Autodesk Inventor part; units mm, degrees
(part 4 of 5)
  arc A1516 (16.6024, 15.6098) -> (16.5463, 15.6184) centre (16.5463, 15.4301) ccw
  arc A1517 (16.6393, 15.5846) -> (16.6024, 15.6098) centre (16.5796, 15.5369) ccw
  arc A1518 (16.6599, 15.5394) -> (16.6393, 15.5846) centre (16.56, 15.5212) ccw
  arc A1519 (16.6663, 15.4684) -> (16.6599, 15.5394) centre (16.2689, 15.4684) ccw
  arc A1520 (16.6599, 14.6174) -> (16.6663, 14.6884) centre (16.2689, 14.6884) ccw
  arc A1521 (16.6393, 14.5721) -> (16.6599, 14.6174) centre (16.56, 14.6356) ccw
  arc A1522 (16.6024, 14.547) -> (16.6393, 14.5721) centre (16.5796, 14.6199) ccw
  arc A1523 (16.5463, 14.5384) -> (16.6024, 14.547) centre (16.5463, 14.7267) ccw
  arc A1524 (16.4902, 14.547) -> (16.5463, 14.5384) centre (16.5463, 14.7267) ccw
  arc A1525 (16.4533, 14.5721) -> (16.4902, 14.547) centre (16.5129, 14.6199) ccw
  arc A1526 (16.4327, 14.6174) -> (16.4533, 14.5721) centre (16.5325, 14.6356) ccw
  arc A1527 (16.4263, 14.6884) -> (16.4327, 14.6174) centre (16.8237, 14.6884) ccw
  arc A1528 (16.4327, 14.7594) -> (16.4263, 14.6884) centre (16.8237, 14.6884) ccw
  arc A1529 (16.4533, 14.8046) -> (16.4327, 14.7594) centre (16.5325, 14.7412) ccw
  arc A1530 (16.4902, 14.8298) -> (16.4533, 14.8046) centre (16.5129, 14.7569) ccw
  arc A1531 (16.5463, 14.8384) -> (16.4902, 14.8298) centre (16.5463, 14.6501) ccw
  arc A1532 (16.6024, 14.8298) -> (16.5463, 14.8384) centre (16.5463, 14.6501) ccw
  arc A1533 (16.6393, 14.8046) -> (16.6024, 14.8298) centre (16.5796, 14.7569) ccw
  arc A1534 (16.6599, 14.7594) -> (16.6393, 14.8046) centre (16.56, 14.7412) ccw
  arc A1535 (16.6663, 14.6884) -> (16.6599, 14.7594) centre (16.2689, 14.6884) ccw
  arc A1536 (16.6306, 13.7177) -> (16.6363, 13.8142) centre (15.8065, 13.8142) ccw
  arc A1537 (16.6121, 13.6524) -> (16.6306, 13.7177) centre (16.4198, 13.7424) ccw
  arc A1538 (16.5793, 13.6115) -> (16.6121, 13.6524) centre (16.5112, 13.6997) ccw
  arc A1539 (16.5313, 13.5898) -> (16.5793, 13.6115) centre (16.5098, 13.7014) ccw
  arc A1540 (16.4797, 13.5909) -> (16.5313, 13.5898) centre (16.508, 13.7107) ccw
  arc A1541 (16.4475, 13.615) -> (16.4797, 13.5909) centre (16.4913, 13.64) ccw
  arc A1542 (16.4306, 13.6695) -> (16.4475, 13.615) centre (16.5623, 13.6804) ccw
  arc A1543 (16.4263, 13.774) -> (16.4306, 13.6695) centre (17.6884, 13.774) ccw
  arc A1544 (16.4293, 13.8553) -> (16.4263, 13.774) centre (17.5205, 13.774) ccw
  arc A1545 (16.4384, 13.9305) -> (16.4293, 13.8553) centre (17.2504, 13.7941) ccw
  arc A1546 (16.4515, 13.9917) -> (16.4384, 13.9305) centre (17.1328, 13.8139) ccw
  arc A1547 (16.4675, 14.0196) -> (16.4515, 13.9917) centre (16.5111, 13.9761) ccw
  arc A1548 (16.5292, 14.0474) -> (16.4675, 14.0196) centre (16.5349, 13.9523) ccw
  arc A1549 (16.5849, 14.0231) -> (16.5292, 14.0474) centre (16.5332, 13.9806) ccw
  arc A1550 (16.6239, 13.9404) -> (16.5849, 14.0231) centre (16.4401, 13.9041) ccw
  arc A1551 (16.6363, 13.8142) -> (16.6239, 13.9404) centre (15.9849, 13.8142) ccw
  arc A1552 (5.9121, 15.2297) -> (5.9567, 15.3581) centre (3.0245, 16.304) ccw
  arc A1553 (5.8608, 15.0999) -> (5.9121, 15.2297) centre (2.705, 16.4228) ccw
  arc A1554 (5.8104, 14.9862) -> (5.8608, 15.0999) centre (3.0618, 16.2733) ccw
  arc A1555 (5.7705, 14.914) -> (5.8104, 14.9862) centre (5.2469, 15.2501) ccw
  arc A1556 (5.7705, 14.914) -> (5.7251, 14.8316) centre (6.3667, 14.5314) ccw
  arc A1557 (5.7251, 14.8316) -> (5.7257, 14.7867) centre (5.7719, 14.8097) ccw
  arc A1558 (5.7257, 14.7867) -> (5.7624, 14.7497) centre (5.8002, 14.8239) ccw
  arc A1559 (5.7624, 14.7497) -> (5.8803, 14.6939) centre (6.7561, 16.6973) ccw
  arc A1560 (5.9708, 14.6449) -> (5.8803, 14.6939) centre (5.6348, 14.1324) ccw
  arc A1561 (5.9663, 14.6196) -> (5.9708, 14.6449) centre (5.9631, 14.6332) ccw
  arc A1562 (5.8708, 14.6078) -> (5.9663, 14.6196) centre (5.8638, 15.0599) ccw
  arc A1563 (5.4913, 14.6033) -> (5.8708, 14.6078) centre (5.0515, 67.172) ccw
  line L488 (5.4913, 14.6033) -> (4.9063, 14.5984)
  line L489 (4.9063, 14.5984) -> (4.9063, 13.4884)
  line L490 (4.9063, 13.4884) -> (4.9063, 12.3784)
  line L491 (4.9063, 12.3784) -> (5.1727, 12.3784)
  arc A1564 (5.1727, 12.3784) -> (5.2775, 12.3828) centre (5.1727, 13.6312) ccw
  arc A1565 (5.2775, 12.3828) -> (5.3718, 12.396) centre (5.206, 13.235) ccw
  arc A1566 (5.3718, 12.396) -> (5.4463, 12.4151) centre (5.2366, 13.0801) ccw
  arc A1567 (5.4463, 12.4151) -> (5.4763, 12.4384) centre (5.4299, 12.4671) ccw
  arc A1568 (5.5036, 12.4616) -> (5.4763, 12.4384) centre (5.5257, 12.4079) ccw
  arc A1569 (5.5621, 12.4808) -> (5.5036, 12.4616) centre (5.6655, 12.0669) ccw
  arc A1570 (5.6359, 12.494) -> (5.5621, 12.4808) centre (5.6964, 11.9435) ccw
  arc A1571 (5.7163, 12.4984) -> (5.6359, 12.494) centre (5.7163, 11.7626) ccw
  arc A1572 (5.7967, 12.494) -> (5.7163, 12.4984) centre (5.7163, 11.7626) ccw
  arc A1573 (5.8705, 12.4808) -> (5.7967, 12.494) centre (5.7362, 11.9435) ccw
  arc A1574 (5.9289, 12.4616) -> (5.8705, 12.4808) centre (5.767, 12.0669) ccw
  arc A1575 (5.9563, 12.4384) -> (5.9289, 12.4616) centre (5.9069, 12.4079) ccw
  arc A1576 (5.9563, 12.4384) -> (5.9863, 12.4151) centre (6.0027, 12.4671) ccw
  arc A1577 (5.9863, 12.4151) -> (6.0607, 12.396) centre (6.196, 13.0801) ccw
  arc A1578 (6.0607, 12.396) -> (6.1551, 12.3828) centre (6.2266, 13.235) ccw
  arc A1579 (6.1551, 12.3828) -> (6.2598, 12.3784) centre (6.2598, 13.6312) ccw
  line L492 (6.2598, 12.3784) -> (6.5263, 12.3784)
  line L493 (6.5263, 12.3784) -> (6.5263, 13.4884)
  line L494 (6.5263, 13.4884) -> (6.5263, 14.5984)
  line L495 (6.5263, 14.5984) -> (6.385, 14.5984)
  line L496 (6.385, 14.5984) -> (6.2438, 14.5984)
  line L497 (6.2438, 14.5984) -> (6.3805, 14.8841)
  arc A1580 (6.3805, 14.8841) -> (6.4343, 15.0063) centre (4.4938, 15.787) ccw
  arc A1581 (6.4343, 15.0063) -> (6.4828, 15.1374) centre (4.1091, 15.9418) ccw
  arc A1582 (6.4828, 15.1374) -> (6.52, 15.2583) centre (4.3654, 15.8549) ccw
  arc A1583 (6.52, 15.2583) -> (6.5368, 15.3451) centre (5.9846, 15.4066) ccw
  arc A1584 (6.5368, 15.3451) -> (6.5386, 15.4464) centre (5.9904, 15.4059) ccw
  arc A1585 (6.5386, 15.4464) -> (6.5135, 15.5043) centre (6.4433, 15.4394) ccw
  arc A1586 (6.5135, 15.5043) -> (6.4513, 15.5459) centre (6.3953, 15.395) ccw
  arc A1587 (6.4513, 15.5459) -> (6.3064, 15.5941) centre (5.6805, 13.471) ccw
  line L498 (6.3064, 15.5941) -> (6.0566, 15.6678)
  line L499 (6.0566, 15.6678) -> (5.9567, 15.3581)
  arc A1588 (5.9784, 13.8303) -> (5.9863, 13.9384) centre (5.2368, 13.9384) ccw
  arc A1589 (5.9488, 13.7834) -> (5.9784, 13.8303) centre (5.9109, 13.8402) ccw
  arc A1590 (5.8854, 13.7625) -> (5.9488, 13.7834) centre (5.8793, 13.8876) ccw
  arc A1591 (5.7163, 13.7584) -> (5.8854, 13.7625) centre (5.7163, 17.2389) ccw
  arc A1592 (5.5472, 13.7625) -> (5.7163, 13.7584) centre (5.7163, 17.2389) ccw
  arc A1593 (5.4838, 13.7834) -> (5.5472, 13.7625) centre (5.5533, 13.8876) ccw
  arc A1594 (5.4541, 13.8303) -> (5.4838, 13.7834) centre (5.5216, 13.8402) ccw
  arc A1595 (5.4463, 13.9384) -> (5.4541, 13.8303) centre (6.1958, 13.9384) ccw
  arc A1596 (5.4541, 14.0465) -> (5.4463, 13.9384) centre (6.1958, 13.9384) ccw
  arc A1597 (5.4838, 14.0934) -> (5.4541, 14.0465) centre (5.5216, 14.0366) ccw
  arc A1598 (5.5472, 14.1143) -> (5.4838, 14.0934) centre (5.5533, 13.9892) ccw
  arc A1599 (5.7163, 14.1184) -> (5.5472, 14.1143) centre (5.7163, 10.6379) ccw
  arc A1600 (5.8854, 14.1143) -> (5.7163, 14.1184) centre (5.7163, 10.6379) ccw
  arc A1601 (5.9488, 14.0934) -> (5.8854, 14.1143) centre (5.8793, 13.9892) ccw
  arc A1602 (5.9784, 14.0465) -> (5.9488, 14.0934) centre (5.9109, 14.0366) ccw
  arc A1603 (5.9863, 13.9384) -> (5.9784, 14.0465) centre (5.2368, 13.9384) ccw
  arc A1604 (5.9795, 12.9829) -> (5.9863, 13.0949) centre (5.0516, 13.0949) ccw
  arc A1605 (5.9519, 12.9387) -> (5.9795, 12.9829) centre (5.9186, 12.9902) ccw
  arc A1606 (5.8934, 12.9222) -> (5.9519, 12.9387) centre (5.8958, 13.0254) ccw
  arc A1607 (5.7313, 12.9299) -> (5.8934, 12.9222) centre (5.9734, 16.2763) ccw
  arc A1608 (5.5847, 12.9458) -> (5.7313, 12.9299) centre (5.8816, 15.0074) ccw
  arc A1609 (5.5151, 12.9725) -> (5.5847, 12.9458) centre (5.6086, 13.1122) ccw
  arc A1610 (5.4776, 13.0216) -> (5.5151, 12.9725) centre (5.5682, 13.0518) ccw
  arc A1611 (5.4573, 13.1134) -> (5.4776, 13.0216) centre (5.9087, 13.1653) ccw
  arc A1612 (5.4541, 13.212) -> (5.4573, 13.1134) centre (6.0551, 13.1822) ccw
  arc A1613 (5.4791, 13.2554) -> (5.4541, 13.212) centre (5.509, 13.2092) ccw
  arc A1614 (5.5401, 13.2748) -> (5.4791, 13.2554) centre (5.5452, 13.1534) ccw
  arc A1615 (5.7123, 13.2784) -> (5.5401, 13.2748) centre (5.7123, 9.1613) ccw
  arc A1616 (5.8852, 13.2743) -> (5.7123, 13.2784) centre (5.7123, 9.5941) ccw
  arc A1617 (5.9489, 13.2534) -> (5.8852, 13.2743) centre (5.8794, 13.1495) ccw
  arc A1618 (5.9786, 13.206) -> (5.9489, 13.2534) centre (5.9108, 13.1965) ccw
  arc A1619 (5.9863, 13.0949) -> (5.9786, 13.206) centre (5.1834, 13.0949) ccw
  arc A1620 (5.1763, 15.5756) -> (5.0533, 15.5279) centre (5.2917, 15.0958) ccw
  arc A1621 (5.0533, 15.5279) -> (4.9985, 15.4587) centre (5.1085, 15.428) ccw
  arc A1622 (4.9985, 15.4587) -> (4.9964, 15.3478) centre (5.2114, 15.3992) ccw
  arc A1623 (4.9964, 15.3478) -> (5.0551, 15.1421) centre (7.4152, 15.926) ccw
  line L500 (5.0551, 15.1421) -> (5.1571, 14.835)
  line L501 (5.1571, 14.835) -> (5.3767, 14.8746)
  arc A1624 (5.3767, 14.8746) -> (5.4626, 14.8914) centre (4.8255, 17.9263) ccw
  arc A1625 (5.4626, 14.8914) -> (5.539, 14.909) centre (5.0517, 16.8488) ccw
  arc A1626 (5.539, 14.909) -> (5.6021, 14.9258) centre (4.9452, 17.2724) ccw
  arc A1627 (5.6021, 14.9258) -> (5.6209, 14.936) centre (5.5891, 14.9722) ccw
  arc A1628 (5.6209, 14.936) -> (5.6282, 14.9553) centre (5.6064, 14.9526) ccw
  arc A1629 (5.6282, 14.9553) -> (5.6151, 15.0484) centre (2.1377, 14.5092) ccw
  arc A1630 (5.6151, 15.0484) -> (5.5949, 15.1599) centre (3.3594, 14.6987) ccw
  arc A1631 (5.5949, 15.1599) -> (5.5664, 15.2881) centre (1.5733, 14.3301) ccw
  arc A1632 (5.5664, 15.2881) -> (5.5061, 15.5023) centre (2.7572, 14.6142) ccw
  arc A1633 (5.5061, 15.5023) -> (5.4474, 15.5839) centre (5.3502, 15.4519) ccw
  arc A1634 (5.4474, 15.5839) -> (5.3578, 15.6077) centre (5.3723, 15.4819) ccw
  arc A1635 (5.3578, 15.6077) -> (5.1763, 15.5756) centre (5.5306, 14.1027) ccw
  arc A1636 (4.3963, 15.4254) -> (4.3262, 15.4003) centre (6.5047, 9.4466) ccw
  arc A1637 (4.3262, 15.4003) -> (4.2648, 15.3772) centre (5.6457, 11.7944) ccw
  arc A1638 (4.2648, 15.3772) -> (4.213, 15.357) centre (6.5581, 9.4269) ccw
  arc A1639 (4.213, 15.357) -> (4.2015, 15.3504) centre (4.2301, 15.3138) ccw
  arc A1640 (4.2015, 15.3504) -> (4.1907, 15.3135) centre (4.2217, 15.3244) ccw
  arc A1641 (4.1907, 15.3135) -> (4.2846, 15.0531) centre (22.7751, 21.87) ccw
  arc A1642 (4.2846, 15.0531) -> (4.3805, 14.801) centre (16.5632, 19.5799) ccw
  arc A1643 (4.3805, 14.801) -> (4.4225, 14.7507) centre (4.477, 14.8389) ccw
  arc A1644 (4.4225, 14.7507) -> (4.5215, 14.7338) centre (4.493, 14.8648) ccw
  arc A1645 (4.5215, 14.7338) -> (4.7003, 14.7868) centre (4.2534, 15.9649) ccw
  arc A1646 (4.7003, 14.7868) -> (4.8621, 14.8621) centre (4.2659, 15.9319) ccw
  arc A1647 (4.8621, 14.8621) -> (4.8854, 14.9263) centre (4.8367, 14.9076) ccw
  arc A1648 (4.8691, 14.9718) -> (4.8854, 14.9263) centre (5.8374, 15.2916) ccw
  arc A1649 (4.8421, 15.0549) -> (4.8691, 14.9718) centre (13.9102, 17.9581) ccw
  arc A1650 (4.8115, 15.152) -> (4.8421, 15.0549) centre (14.7921, 18.2404) ccw
  arc A1651 (4.7811, 15.2522) -> (4.8115, 15.152) centre (15.9198, 18.5894) ccw
  arc A1652 (4.7811, 15.2522) -> (4.7226, 15.4152) centre (3.2292, 14.7872) ccw
  arc A1653 (4.7226, 15.4152) -> (4.665, 15.4742) centre (4.6187, 15.3715) ccw
  arc A1654 (4.665, 15.4742) -> (4.5792, 15.4814) centre (4.6118, 15.3562) ccw
  arc A1655 (4.5792, 15.4814) -> (4.3963, 15.4254) centre (5.1542, 13.2763) ccw
  line L502 (17.3863, 11.5084) -> (17.3863, 11.3584)
  line L503 (17.3863, 11.3584) -> (16.6063, 11.3584)
  line L504 (16.6063, 11.3584) -> (15.8263, 11.3584)
  line L505 (15.8263, 11.3584) -> (15.8263, 10.8784)
  line L506 (15.8263, 10.8784) -> (15.8263, 10.3984)
  line L507 (15.8263, 10.3984) -> (16.1263, 10.3984)
  arc A1656 (16.1263, 10.3984) -> (16.3183, 10.4021) centre (16.1263, 15.337) ccw
  arc A1657 (16.3183, 10.4021) -> (16.3863, 10.4224) centre (16.3127, 10.545) ccw
  arc A1658 (16.3863, 10.4224) -> (16.4178, 10.4692) centre (16.352, 10.4795) ccw
  arc A1659 (16.4178, 10.4692) -> (16.4263, 10.5784) centre (15.718, 10.5784) ccw
  line L508 (16.4263, 10.5784) -> (16.4263, 10.7584)
  line L509 (16.4263, 10.7584) -> (16.7863, 10.7584)
  arc A1660 (17.0333, 10.7493) -> (16.7863, 10.7584) centre (16.7863, 7.3979) ccw
  arc A1661 (17.1238, 10.706) -> (17.0333, 10.7493) centre (17.0232, 10.612) ccw
  arc A1662 (17.1512, 10.6177) -> (17.1238, 10.706) centre (17.0463, 10.6336) ccw
  arc A1663 (17.1085, 10.4134) -> (17.1512, 10.6177) centre (15.2977, 10.8987) ccw
  arc A1664 (17.0633, 10.3374) -> (17.1085, 10.4134) centre (16.9508, 10.4557) ccw
  arc A1665 (16.9858, 10.2973) -> (17.0633, 10.3374) centre (16.9558, 10.4504) ccw
  arc A1666 (16.8319, 10.2813) -> (16.9858, 10.2973) centre (16.8197, 11.1452) ccw
  arc A1667 (16.4193, 10.2784) -> (16.8319, 10.2813) centre (16.4193, 39.5826) ccw
  line L510 (16.4193, 10.2784) -> (15.7663, 10.2784)
  line L511 (15.7663, 10.2784) -> (15.7663, 9.9784)
  line L512 (15.7663, 9.9784) -> (15.7663, 9.6784)
  line L513 (15.7663, 9.6784) -> (16.3063, 9.6784)
  arc A1668 (16.5317, 9.6744) -> (16.3063, 9.6784) centre (16.3063, 3.2633) ccw
  arc A1669 (16.7015, 9.6617) -> (16.5317, 9.6744) centre (16.4568, 7.5438) ccw
  arc A1670 (16.8239, 9.643) -> (16.7015, 9.6617) centre (16.5035, 7.9482) ccw
  arc A1671 (16.8463, 9.616) -> (16.8239, 9.643) centre (16.8188, 9.616) ccw
  arc A1672 (16.7656, 9.369) -> (16.8463, 9.616) centre (16.4279, 9.616) ccw
  arc A1673 (16.4245, 8.9438) -> (16.7656, 9.369) centre (11.8154, 12.9907) ccw
  arc A1674 (16.0426, 8.5495) -> (16.4245, 8.9438) centre (12.1999, 12.6532) ccw
  arc A1675 (15.7692, 8.3893) -> (16.0426, 8.5495) centre (15.5522, 9.0732) ccw
  arc A1676 (15.7692, 8.3893) -> (15.712, 8.3563) centre (15.8159, 8.2423) ccw
  arc A1677 (15.712, 8.3563) -> (15.7, 8.3129) centre (15.7404, 8.3251) ccw
  arc A1678 (15.7, 8.3129) -> (15.736, 8.2395) centre (15.9425, 8.3863) ccw
  arc A1679 (15.736, 8.2395) -> (15.8706, 8.0548) centre (23.8093, 13.9816) ccw
  arc A1680 (15.8706, 8.0548) -> (15.9586, 7.9412) centre (19.1235, 10.4833) ccw
  arc A1681 (15.9586, 7.9412) -> (16.0397, 7.8455) centre (17.8083, 9.427) ccw
  arc A1682 (16.0397, 7.8455) -> (16.1101, 7.7693) centre (18.4082, 9.9635) ccw
  arc A1683 (16.1101, 7.7693) -> (16.1357, 7.7584) centre (16.1357, 7.7938) ccw
  arc A1684 (16.1357, 7.7584) -> (16.1639, 7.7683) centre (16.1357, 7.8036) ccw
  arc A1685 (16.1639, 7.7683) -> (16.2724, 7.8564) centre (10.8985, 14.366) ccw
  arc A1686 (16.2724, 7.8564) -> (16.3985, 7.9641) centre (13.1828, 11.5989) ccw
  arc A1687 (16.3985, 7.9641) -> (16.5397, 8.092) centre (10.815, 14.2754) ccw
  arc A1688 (16.5397, 8.092) -> (16.8123, 8.3769) centre (14.3349, 10.4735) ccw
  arc A1689 (16.8123, 8.3769) -> (17.0755, 8.719) centre (13.2627, 11.3809) ccw
  arc A1690 (17.0755, 8.719) -> (17.301, 9.0767) centre (13.3872, 11.2939) ccw
  arc A1691 (17.301, 9.0767) -> (17.4588, 9.4084) centre (15.0608, 10.3458) ccw
  arc A1692 (17.5024, 9.5018) -> (17.4588, 9.4084) centre (18.2051, 9.1167) ccw
  arc A1693 (17.5558, 9.584) -> (17.5024, 9.5018) centre (18.079, 9.1858) ccw
  arc A1694 (17.6107, 9.6452) -> (17.5558, 9.584) centre (17.9592, 9.277) ccw
  arc A1695 (17.6574, 9.6693) -> (17.6107, 9.6452) centre (17.676, 9.5762) ccw
  arc A1696 (17.7197, 9.6288) -> (17.6574, 9.6693) centre (17.6678, 9.6173) ccw
  arc A1697 (17.7166, 9.5041) -> (17.7197, 9.6288) centre (17.4678, 9.5727) ccw
  arc A1698 (17.627, 9.257) -> (17.7166, 9.5041) centre (16.1086, 9.9473) ccw
  arc A1699 (17.4284, 8.8384) -> (17.627, 9.257) centre (4.6664, 15.1483) ccw
  arc A1700 (17.2717, 8.5317) -> (17.4284, 8.8384) centre (5.8027, 14.5865) ccw
  arc A1701 (17.1842, 8.4028) -> (17.2717, 8.5317) centre (16.6476, 8.8612) ccw
  arc A1702 (17.0976, 8.3397) -> (17.1842, 8.4028) centre (17.0083, 8.553) ccw
  arc A1703 (16.9765, 8.3092) -> (17.0976, 8.3397) centre (16.9367, 8.7242) ccw
  arc A1704 (16.9765, 8.3092) -> (16.8804, 8.2957) centre (17.0797, 7.2327) ccw
  arc A1705 (16.8804, 8.2957) -> (16.8281, 8.2744) centre (16.9064, 8.1568) ccw
  arc A1706 (16.8281, 8.2744) -> (16.8074, 8.2428) centre (16.8548, 8.2342) ccw
  arc A1707 (16.8074, 8.2428) -> (16.8115, 8.1993) centre (16.8871, 8.2284) ccw
  arc A1708 (16.8249, 8.1526) -> (16.8115, 8.1993) centre (16.5504, 8.0992) ccw
  arc A1709 (16.836, 8.0838) -> (16.8249, 8.1526) centre (15.7203, 7.9377) ccw
  arc A1710 (16.8437, 8.0072) -> (16.836, 8.0838) centre (15.582, 7.9195) ccw
  arc A1711 (16.8463, 7.9335) -> (16.8437, 8.0072) centre (15.7829, 7.9335) ccw
  arc A1712 (16.8463, 7.9335) -> (16.854, 7.8299) centre (17.5406, 7.9335) ccw
  arc A1713 (16.854, 7.8299) -> (16.883, 7.7838) centre (16.9214, 7.8401) ccw
  arc A1714 (16.883, 7.7838) -> (16.9444, 7.7632) centre (16.9504, 7.8826) ccw
  arc A1715 (16.9444, 7.7632) -> (17.1013, 7.7596) centre (17.0879, 10.6231) ccw
  arc A1716 (17.1013, 7.7596) -> (17.2475, 7.7651) centre (17.0909, 9.9764) ccw
  arc A1717 (17.2475, 7.7651) -> (17.5193, 7.786) centre (15.6259, 30.6604) ccw
  arc A1718 (17.5193, 7.786) -> (17.8375, 7.8144) centre (15.4614, 32.6484) ccw
  arc A1719 (17.8375, 7.8144) -> (18.1663, 7.8477) centre (15.1144, 36.2745) ccw
  arc A1720 (18.686, 7.9009) -> (18.1663, 7.8477) centre (23.7835, -44.4739) ccw
  arc A1721 (18.8788, 7.907) -> (18.686, 7.9009) centre (18.8286, 6.4353) ccw
  arc A1722 (18.9859, 7.8815) -> (18.8788, 7.907) centre (18.8693, 7.6297) ccw
  arc A1723 (19.0663, 7.8171) -> (18.9859, 7.8815) centre (18.8957, 7.6865) ccw
  arc A1724 (19.0663, 7.8171) -> (19.1278, 7.7518) centre (19.4145, 8.0835) ccw
  arc A1725 (19.1278, 7.7518) -> (19.1781, 7.7372) centre (19.1688, 7.7992) ccw
  arc A1726 (19.1781, 7.7372) -> (19.2451, 7.7618) centre (19.1519, 7.9119) ccw
  arc A1727 (19.2451, 7.7618) -> (19.4118, 7.8687) centre (15.7227, 13.438) ccw
  line L514 (19.4118, 7.8687) -> (19.6674, 8.038)
  line L515 (19.6674, 8.038) -> (19.3711, 8.4532)
  arc A1728 (19.3711, 8.4532) -> (19.2472, 8.6249) centre (3.8221, -2.6409) ccw
  arc A1729 (19.2472, 8.6249) -> (19.1199, 8.7973) centre (3.0308, -3.2188) ccw
  arc A1730 (19.1199, 8.7973) -> (19.006, 8.9481) centre (4.7814, -1.9114) ccw
  arc A1731 (19.006, 8.9481) -> (18.9317, 9.0416) centre (16.5615, 7.0819) ccw
  line L516 (18.9317, 9.0416) -> (18.7885, 9.2148)
  line L517 (18.7885, 9.2148) -> (18.5383, 9.0492)
  line L518 (18.5383, 9.0492) -> (18.288, 8.8836)
  line L519 (18.288, 8.8836) -> (18.4372, 8.7064)
  arc A1732 (18.5553, 8.5548) -> (18.4372, 8.7064) centre (16.4948, 7.072) ccw
  arc A1733 (18.577, 8.4765) -> (18.5553, 8.5548) centre (18.4597, 8.486) ccw
  arc A1734 (18.5376, 8.4315) -> (18.577, 8.4765) centre (18.5271, 8.4805) ccw
  arc A1735 (18.4138, 8.4184) -> (18.5376, 8.4315) centre (18.4138, 9.0089) ccw
  arc A1736 (18.4138, 8.4184) -> (18.3339, 8.4157) centre (18.4138, 7.253) ccw
  arc A1737 (18.3339, 8.4157) -> (18.2353, 8.4071) centre (18.5194, 5.7156) ccw
  arc A1738 (18.2353, 8.4071) -> (18.1348, 8.3946) centre (18.5277, 5.637) ccw
  arc A1739 (18.1348, 8.3946) -> (18.0484, 8.3798) centre (18.3562, 6.8412) ccw
  line L520 (18.0484, 8.3798) -> (17.8556, 8.3413)
  line L521 (17.8556, 8.3413) -> (18.0379, 8.6648)
  arc A1740 (18.0379, 8.6648) -> (18.1147, 8.8053) centre (12.7688, 11.6345) ccw
  arc A1741 (18.1147, 8.8053) -> (18.1945, 8.96) centre (10.6501, 12.7558) ccw
  arc A1742 (18.1945, 8.96) -> (18.2659, 9.1057) centre (11.242, 12.458) ccw
  arc A1743 (18.2659, 9.1057) -> (18.3148, 9.2152) centre (16.1154, 10.132) ccw
  line L522 (18.3148, 9.2152) -> (18.4094, 9.442)
  line L523 (18.4094, 9.442) -> (18.1528, 9.556)
  line L524 (18.1528, 9.556) -> (17.8963, 9.6699)
  line L525 (17.8963, 9.6699) -> (18.7813, 9.6742)
  line L526 (18.7813, 9.6742) -> (19.6663, 9.6784)
  line L527 (19.6663, 9.6784) -> (19.6663, 9.9784)
  line L528 (19.6663, 9.9784) -> (19.6663, 10.2784)
  line L529 (19.6663, 10.2784) -> (18.7015, 10.2784)
  line L530 (18.7015, 10.2784) -> (17.7367, 10.2784)
  line L531 (17.7367, 10.2784) -> (17.7758, 10.4562)
  arc A1744 (17.7758, 10.4562) -> (17.7925, 10.5737) centre (16.9996, 10.6267) ccw
  arc A1745 (17.7925, 10.5737) -> (17.7687, 10.6248) centre (17.7342, 10.5776) ccw
  arc A1746 (17.7687, 10.6248) -> (17.6976, 10.6572) centre (17.6546, 10.4688) ccw
  arc A1747 (17.6976, 10.6572) -> (17.4163, 10.7191) centre (13.7072, -6.8208) ccw
  arc A1748 (17.417, 10.7294) -> (17.4163, 10.7191) centre (17.4174, 10.7242) ccw
  arc A1749 (17.5827, 10.7391) -> (17.417, 10.7294) centre (17.8361, 4.9792) ccw
  arc A1750 (17.8313, 10.747) -> (17.5827, 10.7391) centre (18.0331, 0.5019) ccw
  arc A1751 (18.1513, 10.7514) -> (17.8313, 10.747) centre (18.3767, -16.9428) ccw
  line L532 (18.1513, 10.7514) -> (19.0063, 10.7584)
  line L533 (19.0063, 10.7584) -> (19.0063, 10.5784)
  arc A1752 (19.0063, 10.5784) -> (19.0147, 10.4692) centre (19.7146, 10.5784) ccw
  arc A1753 (19.0147, 10.4692) -> (19.0463, 10.4224) centre (19.0805, 10.4795) ccw
  arc A1754 (19.0463, 10.4224) -> (19.1143, 10.4021) centre (19.1198, 10.545) ccw
  arc A1755 (19.1143, 10.4021) -> (19.3063, 10.3984) centre (19.3063, 15.337) ccw
  line L534 (19.3063, 10.3984) -> (19.6063, 10.3984)
  line L535 (19.6063, 10.3984) -> (19.6063, 10.8784)
  line L536 (19.6063, 10.8784) -> (19.6063, 11.3584)
  line L537 (19.6063, 11.3584) -> (18.7963, 11.3584)
  line L538 (18.7963, 11.3584) -> (17.9863, 11.3584)
  line L539 (17.9863, 11.3584) -> (17.9863, 11.5084)
  arc A1756 (17.9863, 11.5084) -> (17.9755, 11.5936) centre (17.645, 11.5084) ccw
  arc A1757 (17.9755, 11.5936) -> (17.9413, 11.6359) centre (17.9119, 11.5772) ccw
  arc A1758 (17.9413, 11.6359) -> (17.8687, 11.6546) centre (17.8613, 11.4759) ccw
  arc A1759 (17.8687, 11.6546) -> (17.6863, 11.6584) centre (17.6863, 7.2405) ccw
  arc A1760 (17.6863, 11.6584) -> (17.5039, 11.6546) centre (17.6863, 7.2405) ccw
  arc A1761 (17.5039, 11.6546) -> (17.4313, 11.6359) centre (17.5113, 11.4759) ccw
  arc A1762 (17.4313, 11.6359) -> (17.3971, 11.5936) centre (17.4606, 11.5772) ccw
  arc A1763 (17.3971, 11.5936) -> (17.3863, 11.5084) centre (17.7275, 11.5084) ccw
  arc A1764 (21.734, 11.4718) -> (21.7663, 11.5384) centre (21.6815, 11.5384) ccw
  arc A1765 (21.65, 11.4356) -> (21.734, 11.4718) centre (21.624, 11.6114) ccw
  arc A1766 (21.4644, 11.421) -> (21.65, 11.4356) centre (21.4505, 12.7826) ccw
  arc A1767 (20.9563, 11.4184) -> (21.4644, 11.421) centre (20.9562, 61.232) ccw
  line L540 (20.9563, 11.4184) -> (20.1463, 11.4184)
  line L541 (20.1463, 11.4184) -> (20.1463, 11.1484)
  line L542 (20.1463, 11.1484) -> (20.1463, 10.8784)
  line L543 (20.1463, 10.8784) -> (20.9563, 10.8784)
  arc A1768 (21.294, 10.8746) -> (20.9563, 10.8784) centre (20.9563, -4.0944) ccw
  arc A1769 (21.5488, 10.8623) -> (21.294, 10.8746) centre (21.182, 5.9112) ccw
  arc A1770 (21.7424, 10.8449) -> (21.5488, 10.8623) centre (21.0891, 4.6567) ccw
  arc A1771 (21.7663, 10.8184) -> (21.7424, 10.8449) centre (21.7396, 10.8184) ccw
  arc A1772 (21.7442, 10.7928) -> (21.7663, 10.8184) centre (21.7404, 10.8184) ccw
  arc A1773 (21.6013, 10.7749) -> (21.7442, 10.7928) centre (21.3134, 13.654) ccw
  arc A1774 (21.4112, 10.7623) -> (21.6013, 10.7749) centre (21.3202, 13.5861) ccw
  arc A1775 (21.1663, 10.7584) -> (21.4112, 10.7623) centre (21.1663, 18.3605) ccw
  line L544 (21.1663, 10.7584) -> (20.5663, 10.7584)
  line L545 (20.5663, 10.7584) -> (20.5663, 9.8884)
  line L546 (20.5663, 9.8884) -> (20.5663, 9.0184)
  line L547 (20.5663, 9.0184) -> (21.2898, 9.0184)
  arc A1776 (21.5715, 9.0147) -> (21.2898, 9.0184) centre (21.2898, -1.6524) ccw
  arc A1777 (21.7962, 9.003) -> (21.5715, 9.0147) centre (21.4558, 4.6312) ccw
  arc A1778 (21.9694, 8.9867) -> (21.7962, 9.003) centre (21.3777, 3.6289) ccw
  arc A1779 (21.9801, 8.9646) -> (21.9694, 8.9867) centre (21.9678, 8.9723) ccw
  arc A1780 (21.9801, 8.9646) -> (21.9729, 8.933) centre (22.0228, 8.9383) ccw
  arc A1781 (21.9729, 8.933) -> (21.9829, 8.8764) centre (22.3831, 8.9761) ccw
  arc A1782 (21.9829, 8.8764) -> (22.0045, 8.8091) centre (22.5019, 9.0057) ccw
  arc A1783 (22.0045, 8.8091) -> (22.0362, 8.7396) centre (22.6859, 9.0785) ccw
  arc A1784 (22.0704, 8.6681) -> (22.0362, 8.7396) centre (21.0214, 8.2103) ccw
  arc A1785 (22.0994, 8.5948) -> (22.0704, 8.6681) centre (21.0446, 8.2205) ccw
  arc A1786 (22.12, 8.5294) -> (22.0994, 8.5948) centre (21.1863, 8.2708) ccw
  arc A1787 (22.1259, 8.4869) -> (22.12, 8.5294) centre (21.964, 8.4862) ccw
  arc A1788 (22.1259, 8.4869) -> (22.1532, 8.446) centre (22.1705, 8.4871) ccw
  arc A1789 (22.1532, 8.446) -> (22.2232, 8.4345) centre (22.2123, 8.5866) ccw
  arc A1790 (22.2232, 8.4345) -> (22.3414, 8.4564) centre (22.1845, 8.9724) ccw
  arc A1791 (22.3414, 8.4564) -> (22.5107, 8.5146) centre (21.6115, 10.8578) ccw
  arc A1792 (22.5713, 8.5258) -> (22.5107, 8.5146) centre (22.5711, 8.3572) ccw
  arc A1793 (22.6011, 8.5037) -> (22.5713, 8.5258) centre (22.5713, 8.4945) ccw
  arc A1794 (22.5981, 8.4516) -> (22.6011, 8.5037) centre (22.5293, 8.4817) ccw
  arc A1795 (22.5549, 8.3703) -> (22.5981, 8.4516) centre (22.0465, 8.6928) ccw
  arc A1796 (22.511, 8.3357) -> (22.5549, 8.3703) centre (22.4837, 8.4154) ccw
  arc A1797 (22.4251, 8.3152) -> (22.511, 8.3357) centre (22.3622, 8.77) ccw
  arc A1798 (22.2988, 8.3064) -> (22.4251, 8.3152) centre (22.2961, 9.2487) ccw
  arc A1799 (22.1208, 8.3103) -> (22.2988, 8.3064) centre (22.2884, 11.8682) ccw
  line L548 (22.1208, 8.3103) -> (21.7363, 8.3284)
  line L549 (21.7363, 8.3284) -> (21.7181, 8.6434)
  line L550 (21.7181, 8.6434) -> (21.7, 8.9584)
  line L551 (21.7, 8.9584) -> (21.4331, 8.9584)
  line L552 (21.4331, 8.9584) -> (21.1663, 8.9584)
  line L553 (21.1663, 8.9584) -> (21.1663, 8.4577)
  arc A1800 (21.1663, 8.4577) -> (21.1903, 8.0214) centre (25.1452, 8.4577) ccw
  arc A1801 (21.1903, 8.0214) -> (21.2908, 7.8486) centre (21.4355, 8.0484) ccw
  arc A1802 (21.2908, 7.8486) -> (21.5083, 7.7728) centre (21.5261, 8.1737) ccw
  arc A1803 (21.5083, 7.7728) -> (22.131, 7.7593) centre (22.1142, 21.4134) ccw
  arc A1804 (22.131, 7.7593) -> (22.4218, 7.763) centre (22.1152, 20.5491) ccw
  arc A1805 (22.4218, 7.763) -> (22.6784, 7.7734) centre (22.2347, 15.5653) ccw
  arc A1806 (22.6784, 7.7734) -> (22.8933, 7.7876) centre (22.0328, 19.1107) ccw
  arc A1807 (22.8933, 7.7876) -> (22.948, 7.8058) centre (22.8843, 7.9061) ccw
  arc A1808 (22.948, 7.8058) -> (22.9825, 7.8391) centre (22.8836, 7.9072) ccw
  arc A1809 (22.9825, 7.8391) -> (23.0322, 7.9169) centre (21.8627, 8.6093) ccw
  arc A1810 (23.0322, 7.9169) -> (23.085, 8.0138) centre (21.7118, 8.6986) ccw
  arc A1811 (23.085, 8.0138) -> (23.134, 8.1199) centre (21.354, 8.8771) ccw
  line L554 (23.134, 8.1199) -> (23.2482, 8.3884)
  line L555 (23.2482, 8.3884) -> (23.3784, 8.1334)
  arc A1812 (23.3784, 8.1334) -> (23.4315, 8.0359) centre (25.2609, 9.0951) ccw
  arc A1813 (23.4315, 8.0359) -> (23.4833, 7.9541) centre (24.4912, 8.6495) ccw
  arc A1814 (23.4833, 7.9541) -> (23.5294, 7.8915) centre (24.5333, 8.6785) ccw
  arc A1815 (23.5294, 7.8915) -> (23.5525, 7.8811) centre (23.5508, 7.9083) ccw
  arc A1816 (23.5525, 7.8811) -> (23.5805, 7.8878) centre (23.5473, 7.9651) ccw
  arc A1817 (23.5805, 7.8878) -> (23.6576, 7.9219) centre (22.0711, 11.405) ccw
  arc A1818 (23.6576, 7.9219) -> (23.7489, 7.9652) centre (22.3378, 10.8196) ccw
  arc A1819 (23.7489, 7.9652) -> (23.8489, 8.0161) centre (21.6131, 12.2854) ccw
  line L556 (23.8489, 8.0161) -> (24.1015, 8.1484)
  line L557 (24.1015, 8.1484) -> (23.9389, 8.4212)
  arc A1820 (23.9389, 8.4212) -> (23.7054, 8.8032) centre (6.5644, -1.9355) ccw
  arc A1821 (23.7054, 8.8032) -> (23.6076, 8.9059) centre (23.4048, 8.6149) ccw
  arc A1822 (23.6076, 8.9059) -> (23.5009, 8.927) centre (23.5303, 8.795) ccw
  arc A1823 (23.5009, 8.927) -> (23.2996, 8.8665) centre (23.8145, 7.5184) ccw
  arc A1824 (23.2996, 8.8665) -> (23.1523, 8.8052) centre (24.2748, 6.3129) ccw
  arc A1825 (23.1523, 8.8052) -> (23.0824, 8.7583) centre (23.2557, 8.5756) ccw
  arc A1826 (23.0824, 8.7583) -> (23.0562, 8.7074) centre (23.1421, 8.6954) ccw
  arc A1827 (23.0562, 8.7074) -> (23.0618, 8.641) centre (23.2055, 8.6866) ccw
  arc A1828 (23.0779, 8.576) -> (23.0618, 8.641) centre (22.5665, 8.4838) ccw
  arc A1829 (23.0678, 8.5491) -> (23.0779, 8.576) centre (23.0504, 8.571) ccw
  arc A1830 (23.0365, 8.5413) -> (23.0678, 8.5491) centre (23.0434, 8.5798) ccw
  arc A1831 (22.9581, 8.5588) -> (23.0365, 8.5413) centre (23.2086, 9.4947) ccw
  arc A1832 (22.9581, 8.5588) -> (22.901, 8.5734) centre (22.2799, 6.0253) ccw
  arc A1833 (22.901, 8.5734) -> (22.8468, 8.5858) centre (22.4067, 6.5454) ccw
  arc A1834 (22.8468, 8.5858) -> (22.8008, 8.5952) centre (22.4252, 6.6309) ccw
  arc A1835 (22.8008, 8.5952) -> (22.7783, 8.5976) centre (22.7754, 8.462) ccw
  arc A1836 (22.7616, 8.6049) -> (22.7783, 8.5976) centre (22.7788, 8.6214) ccw
  arc A1837 (22.7426, 8.629) -> (22.7616, 8.6049) centre (22.877, 8.7156) ccw
  arc A1838 (22.7244, 8.6631) -> (22.7426, 8.629) centre (22.9363, 8.7538) ccw
  arc A1839 (22.7101, 8.7034) -> (22.7244, 8.6631) centre (23.0401, 8.7983) ccw
  arc A1840 (22.7101, 8.7034) -> (22.6954, 8.7512) centre (21.3706, 8.3183) ccw
  arc A1841 (22.6954, 8.7512) -> (22.6761, 8.8084) centre (19.8918, 7.835) ccw
  arc A1842 (22.6761, 8.8084) -> (22.6554, 8.8656) centre (19.8685, 7.8269) ccw
  arc A1843 (22.6554, 8.8656) -> (22.6367, 8.9134) centre (21.2304, 8.3345) ccw
  arc A1844 (22.6392, 8.9682) -> (22.6367, 8.9134) centre (22.6966, 8.9381) ccw
  arc A1845 (22.683, 9.0016) -> (22.6392, 8.9682) centre (22.6971, 8.9378) ccw
  arc A1846 (22.8023, 9.0157) -> (22.683, 9.0016) centre (22.8127, 8.4169) ccw
  arc A1847 (23.1099, 9.0184) -> (22.8023, 9.0157) centre (23.1099, -8.7429) ccw
  line L558 (23.1099, 9.0184) -> (23.6263, 9.0184)
  line L559 (23.6263, 9.0184) -> (23.6263, 9.8884)
  line L560 (23.6263, 9.8884) -> (23.6263, 10.7584)
  line L561 (23.6263, 10.7584) -> (22.9963, 10.7584)
  arc A1848 (22.7381, 10.7623) -> (22.9963, 10.7584) centre (22.9963, 19.2595) ccw
  arc A1849 (22.5388, 10.7748) -> (22.7381, 10.7623) centre (22.8321, 13.8544) ccw
  arc A1850 (22.3886, 10.7926) -> (22.5388, 10.7748) centre (22.8483, 14.0251) ccw
  arc A1851 (22.3663, 10.8184) -> (22.3886, 10.7926) centre (22.3923, 10.8184) ccw
  arc A1852 (22.3903, 10.845) -> (22.3663, 10.8184) centre (22.393, 10.8184) ccw
  arc A1853 (22.5913, 10.8623) -> (22.3903, 10.845) centre (23.0794, 4.029) ccw
  arc A1854 (22.8553, 10.8746) -> (22.5913, 10.8623) centre (22.9703, 5.5558) ccw
  arc A1855 (23.2063, 10.8784) -> (22.8553, 10.8746) centre (23.2063, -5.3532) ccw
  line L562 (23.2063, 10.8784) -> (24.0463, 10.8784)
  line L563 (24.0463, 10.8784) -> (24.0463, 11.1484)
  line L564 (24.0463, 11.1484) -> (24.0463, 11.4184)
  line L565 (24.0463, 11.4184) -> (23.2307, 11.4184)
  arc A1856 (22.7279, 11.4212) -> (23.2307, 11.4184) centre (23.2307, 56.2644) ccw
  arc A1857 (22.5313, 11.4362) -> (22.7279, 11.4212) centre (22.7449, 12.9443) ccw
  arc A1858 (22.4331, 11.4716) -> (22.5313, 11.4362) centre (22.5671, 11.6892) ccw
  arc A1859 (22.3837, 11.5384) -> (22.4331, 11.4716) centre (22.4916, 11.5666) ccw
  arc A1860 (22.3837, 11.5384) -> (22.3531, 11.5993) centre (22.2253, 11.497) ccw
  arc A1861 (22.3531, 11.5993) -> (22.3027, 11.6356) centre (22.2624, 11.5266) ccw
  arc A1862 (22.3027, 11.6356) -> (22.2165, 11.6537) centre (22.1987, 11.3546) ccw
  arc A1863 (22.2165, 11.6537) -> (22.0593, 11.6584) centre (22.0593, 9.0071) ccw
  arc A1864 (22.0593, 11.6584) -> (21.8953, 11.6544) centre (22.0593, 8.2557) ccw
  arc A1865 (21.8953, 11.6544) -> (21.8179, 11.6373) centre (21.9066, 11.4206) ccw
  arc A1866 (21.8179, 11.6373) -> (21.78, 11.601) centre (21.845, 11.571) ccw
  arc A1867 (21.78, 11.601) -> (21.7663, 11.5384) centre (21.9156, 11.5384) ccw
  arc A1868 (21.7486, 10.146) -> (21.7663, 10.1884) centre (21.7066, 10.1884) ccw
  arc A1869 (21.7013, 10.1179) -> (21.7486, 10.146) centre (21.6686, 10.2268) ccw
  arc A1870 (21.6139, 10.1026) -> (21.7013, 10.1179) centre (21.5926, 10.48) ccw
  arc A1871 (21.4663, 10.0984) -> (21.6139, 10.1026) centre (21.4663, 12.7235) ccw
  arc A1872 (21.3186, 10.1026) -> (21.4663, 10.0984) centre (21.4663, 12.7235) ccw
  arc A1873 (21.2313, 10.1179) -> (21.3186, 10.1026) centre (21.3399, 10.48) ccw
  arc A1874 (21.184, 10.146) -> (21.2313, 10.1179) centre (21.2639, 10.2268) ccw
  arc A1875 (21.1663, 10.1884) -> (21.184, 10.146) centre (21.226, 10.1884) ccw
  arc A1876 (21.184, 10.2308) -> (21.1663, 10.1884) centre (21.226, 10.1884) ccw
  arc A1877 (21.2313, 10.2589) -> (21.184, 10.2308) centre (21.2639, 10.15) ccw
  arc A1878 (21.3186, 10.2742) -> (21.2313, 10.2589) centre (21.3399, 9.8968) ccw
  arc A1879 (21.4663, 10.2784) -> (21.3186, 10.2742) centre (21.4663, 7.6533) ccw
  arc A1880 (21.6139, 10.2742) -> (21.4663, 10.2784) centre (21.4663, 7.6533) ccw
  arc A1881 (21.7013, 10.2589) -> (21.6139, 10.2742) centre (21.5926, 9.8968) ccw
  arc A1882 (21.7486, 10.2308) -> (21.7013, 10.2589) centre (21.6686, 10.15) ccw
  arc A1883 (21.7663, 10.1884) -> (21.7486, 10.2308) centre (21.7066, 10.1884) ccw
  arc A1884 (23.0073, 10.1455) -> (23.0263, 10.1884) centre (22.9683, 10.1884) ccw
  arc A1885 (22.9563, 10.1175) -> (23.0073, 10.1455) centre (22.9235, 10.2377) ccw
  arc A1886 (22.8612, 10.1024) -> (22.9563, 10.1175) centre (22.8397, 10.545) ccw
  arc A1887 (22.6963, 10.0984) -> (22.8612, 10.1024) centre (22.6963, 13.5008) ccw
  arc A1888 (22.5314, 10.1024) -> (22.6963, 10.0984) centre (22.6963, 13.5008) ccw
  arc A1889 (22.4363, 10.1175) -> (22.5314, 10.1024) centre (22.5529, 10.545) ccw
  arc A1890 (22.3853, 10.1455) -> (22.4363, 10.1175) centre (22.4691, 10.2377) ccw
  arc A1891 (22.3663, 10.1884) -> (22.3853, 10.1455) centre (22.4243, 10.1884) ccw
  arc A1892 (22.3853, 10.2313) -> (22.3663, 10.1884) centre (22.4243, 10.1884) ccw
  arc A1893 (22.4363, 10.2593) -> (22.3853, 10.2313) centre (22.4691, 10.1391) ccw
  arc A1894 (22.5314, 10.2744) -> (22.4363, 10.2593) centre (22.5529, 9.8318) ccw
  arc A1895 (22.6963, 10.2784) -> (22.5314, 10.2744) centre (22.6963, 6.876) ccw
  arc A1896 (22.8612, 10.2744) -> (22.6963, 10.2784) centre (22.6963, 6.876) ccw
  arc A1897 (22.9563, 10.2593) -> (22.8612, 10.2744) centre (22.8397, 9.8318) ccw
  arc A1898 (23.0073, 10.2313) -> (22.9563, 10.2593) centre (22.9235, 10.1391) ccw
  arc A1899 (23.0263, 10.1884) -> (23.0073, 10.2313) centre (22.9683, 10.1884) ccw
  arc A1900 (21.7486, 9.546) -> (21.7663, 9.5884) centre (21.7066, 9.5884) ccw
  arc A1901 (21.7013, 9.5179) -> (21.7486, 9.546) centre (21.6686, 9.6268) ccw
  arc A1902 (21.6139, 9.5026) -> (21.7013, 9.5179) centre (21.5926, 9.88) ccw
  arc A1903 (21.4663, 9.4984) -> (21.6139, 9.5026) centre (21.4663, 12.1235) ccw
  arc A1904 (21.3186, 9.5026) -> (21.4663, 9.4984) centre (21.4663, 12.1235) ccw
  arc A1905 (21.2313, 9.5179) -> (21.3186, 9.5026) centre (21.3399, 9.88) ccw
  arc A1906 (21.184, 9.546) -> (21.2313, 9.5179) centre (21.2639, 9.6268) ccw
  arc A1907 (21.1663, 9.5884) -> (21.184, 9.546) centre (21.226, 9.5884) ccw
  arc A1908 (21.184, 9.6308) -> (21.1663, 9.5884) centre (21.226, 9.5884) ccw
  arc A1909 (21.2313, 9.6589) -> (21.184, 9.6308) centre (21.2639, 9.55) ccw
  arc A1910 (21.3186, 9.6742) -> (21.2313, 9.6589) centre (21.3399, 9.2968) ccw
  arc A1911 (21.4663, 9.6784) -> (21.3186, 9.6742) centre (21.4663, 7.0533) ccw
  arc A1912 (21.6139, 9.6742) -> (21.4663, 9.6784) centre (21.4663, 7.0533) ccw
  arc A1913 (21.7013, 9.6589) -> (21.6139, 9.6742) centre (21.5926, 9.2968) ccw
  arc A1914 (21.7486, 9.6308) -> (21.7013, 9.6589) centre (21.6686, 9.55) ccw
  arc A1915 (21.7663, 9.5884) -> (21.7486, 9.6308) centre (21.7066, 9.5884) ccw
  arc A1916 (23.0073, 9.5455) -> (23.0263, 9.5884) centre (22.9683, 9.5884) ccw
  arc A1917 (22.9563, 9.5175) -> (23.0073, 9.5455) centre (22.9235, 9.6377) ccw
  arc A1918 (22.8612, 9.5024) -> (22.9563, 9.5175) centre (22.8397, 9.945) ccw
  arc A1919 (22.6963, 9.4984) -> (22.8612, 9.5024) centre (22.6963, 12.9008) ccw
  arc A1920 (22.5314, 9.5024) -> (22.6963, 9.4984) centre (22.6963, 12.9008) ccw
  arc A1921 (22.4363, 9.5175) -> (22.5314, 9.5024) centre (22.5529, 9.945) ccw
  arc A1922 (22.3853, 9.5455) -> (22.4363, 9.5175) centre (22.4691, 9.6377) ccw
  arc A1923 (22.3663, 9.5884) -> (22.3853, 9.5455) centre (22.4243, 9.5884) ccw
  arc A1924 (22.3853, 9.6313) -> (22.3663, 9.5884) centre (22.4243, 9.5884) ccw
  arc A1925 (22.4363, 9.6593) -> (22.3853, 9.6313) centre (22.4691, 9.5391) ccw
  arc A1926 (22.5314, 9.6744) -> (22.4363, 9.6593) centre (22.5529, 9.2318) ccw
  arc A1927 (22.6963, 9.6784) -> (22.5314, 9.6744) centre (22.6963, 6.276) ccw
  arc A1928 (22.8612, 9.6744) -> (22.6963, 9.6784) centre (22.6963, 6.276) ccw
  arc A1929 (22.9563, 9.6593) -> (22.8612, 9.6744) centre (22.8397, 9.2318) ccw
  arc A1930 (23.0073, 9.6313) -> (22.9563, 9.6593) centre (22.9235, 9.5391) ccw
  arc A1931 (23.0263, 9.5884) -> (23.0073, 9.6313) centre (22.9683, 9.5884) ccw
  arc A1932 (20.3482, 8.5997) -> (20.3988, 8.7034) centre (18.968, 9.3378) ccw
  arc A1933 (20.2897, 8.4991) -> (20.3482, 8.5997) centre (18.917, 9.365) ccw
  arc A1934 (20.2319, 8.4145) -> (20.2897, 8.4991) centre (19.0975, 9.2512) ccw
  arc A1935 (20.186, 8.3661) -> (20.2319, 8.4145) centre (20.0122, 8.5766) ccw
  arc A1936 (20.186, 8.3661) -> (20.1106, 8.2779) centre (20.4006, 8.1061) ccw
  arc A1937 (20.1106, 8.2779) -> (20.0984, 8.193) centre (20.2073, 8.2206) ccw
  arc A1938 (20.0984, 8.193) -> (20.1509, 8.0922) centre (20.338, 8.2538) ccw
  arc A1939 (20.1509, 8.0922) -> (20.2938, 7.9408) centre (21.9256, 9.6244) ccw
  arc A1940 (20.2938, 7.9408) -> (20.4088, 7.8355) centre (22.2213, 9.9294) ccw
  arc A1941 (20.4088, 7.8355) -> (20.4794, 7.7915) centre (20.5828, 8.0366) ccw
  arc A1942 (20.4794, 7.7915) -> (20.5356, 7.7868) centre (20.5148, 7.8753) ccw
  arc A1943 (20.5356, 7.7868) -> (20.5921, 7.8149) centre (20.504, 7.921) ccw
  arc A1944 (20.5921, 7.8149) -> (20.688, 7.9295) centre (20.3278, 8.1334) ccw
  arc A1945 (20.688, 7.9295) -> (20.8577, 8.2428) centre (12.3018, 12.6761) ccw
  arc A1946 (20.8577, 8.2428) -> (21.0175, 8.5641) centre (11.2584, 13.2167) ccw
  arc A1947 (21.0175, 8.5641) -> (21.0463, 8.6915) centre (20.7503, 8.6915) ccw
  arc A1948 (21.0463, 8.6915) -> (21.0158, 8.7452) centre (20.9838, 8.6915) ccw
  arc A1949 (21.0158, 8.7452) -> (20.834, 8.8469) centre (19.0328, 5.4163) ccw
  arc A1950 (20.834, 8.8469) -> (20.6478, 8.9357) centre (19.5858, 6.4696) ccw
  arc A1951 (20.6478, 8.9357) -> (20.5379, 8.9584) centre (20.5379, 8.6804) ccw
  arc A1952 (20.5379, 8.9584) -> (20.5239, 8.9504) centre (20.5379, 8.9423) ccw
  arc A1953 (20.5239, 8.9504) -> (20.4863, 8.8835) centre (23.0469, 7.4874) ccw
  arc A1954 (20.4863, 8.8835) -> (20.444, 8.8011) centre (22.112, 7.9971) ccw
  arc A1955 (20.444, 8.8011) -> (20.3988, 8.7034) centre (23.4887, 7.3335) ccw
  arc A1956 (16.104, 6.3417) -> (16.1615, 6.5229) centre (12.9758, 7.4352) ccw
  arc A1957 (16.0234, 6.1223) -> (16.104, 6.3417) centre (9.0107, 8.8214) ccw
  arc A1958 (15.9344, 5.9013) -> (16.0234, 6.1223) centre (8.8454, 8.885) ccw
  arc A1959 (15.8504, 5.7145) -> (15.9344, 5.9013) centre (12.0427, 7.5393) ccw
  line L566 (15.8504, 5.7145) -> (15.6525, 5.3016)
  line L567 (15.6525, 5.3016) -> (15.7593, 4.9873)
  arc A1960 (15.7593, 4.9873) -> (15.8248, 4.8022) centre (23.2048, 7.5181) ccw
  arc A1961 (15.8248, 4.8022) -> (15.8598, 4.7439) centre (15.9962, 4.8653) ccw
  arc A1962 (15.8598, 4.7439) -> (15.8931, 4.7415) centre (15.8777, 4.7598) ccw
  arc A1963 (15.8931, 4.7415) -> (15.9344, 4.7907) centre (15.772, 4.8849) ccw
  arc A1964 (15.9667, 4.7879) -> (15.9344, 4.7907) centre (15.9499, 4.7817) ccw
  arc A1965 (15.9888, 4.6873) -> (15.9667, 4.7879) centre (15.5986, 4.6543) ccw
  arc A1966 (16.0008, 4.4424) -> (15.9888, 4.6873) centre (12.5549, 4.3965) ccw
  arc A1967 (16.0045, 3.9634) -> (16.0008, 4.4424) centre (-26.0177, 3.8823) ccw
  line L568 (16.0045, 3.9634) -> (16.0063, 3.0184)
  line L569 (16.0063, 3.0184) -> (16.2763, 3.0184)
  line L570 (16.2763, 3.0184) -> (16.5463, 3.0184)
  line L571 (16.5463, 3.0184) -> (16.5488, 3.6934)
  line L572 (16.5488, 3.6934) -> (16.5513, 4.3684)
  line L573 (16.5513, 4.3684) -> (16.6663, 4.1584)
  arc A1968 (16.7504, 3.9858) -> (16.6663, 4.1584) centre (14.8949, 3.1886) ccw
  arc A1969 (16.7776, 3.8688) -> (16.7504, 3.9858) centre (16.4375, 3.8514) ccw
  arc A1970 (16.758, 3.7721) -> (16.7776, 3.8688) centre (16.5787, 3.8586) ccw
  arc A1971 (16.6911, 3.6727) -> (16.758, 3.7721) centre (16.3794, 3.9548) ccw
  arc A1972 (16.6911, 3.6727) -> (16.6444, 3.6035) centre (16.9097, 3.4748) ccw
  arc A1973 (16.6444, 3.6035) -> (16.6356, 3.5412) centre (16.7368, 3.5587) ccw
  arc A1974 (16.6356, 3.5412) -> (16.6639, 3.4589) centre (16.9056, 3.5879) ccw
  arc A1975 (16.6639, 3.4589) -> (16.7568, 3.2929) centre (20.8949, 5.718) ccw
  arc A1976 (16.7568, 3.2929) -> (16.8214, 3.1877) centre (19.2997, 4.7832) ccw
  arc A1977 (16.8214, 3.1877) -> (16.8826, 3.099) centre (18.2605, 4.1142) ccw
  arc A1978 (16.8826, 3.099) -> (16.9362, 3.0293) centre (18.5579, 4.3332) ccw
  arc A1979 (16.9362, 3.0293) -> (16.959, 3.0184) centre (16.959, 3.0477) ccw
  arc A1980 (16.959, 3.0184) -> (16.9806, 3.0275) centre (16.959, 3.0485) ccw
  arc A1981 (16.9806, 3.0275) -> (17.0189, 3.0702) centre (16.472, 3.5214) ccw
  arc A1982 (17.0189, 3.0702) -> (17.0617, 3.1273) centre (16.4176, 3.5663) ccw
  arc A1983 (17.0617, 3.1273) -> (17.1046, 3.1949) centre (16.0402, 3.8237) ccw
  line L574 (17.1046, 3.1949) -> (17.2089, 3.3713)
  line L575 (17.2089, 3.3713) -> (17.4926, 3.2284)
  arc A1984 (17.4926, 3.2284) -> (17.6815, 3.1512) centre (18.0787, 4.3923) ccw
  arc A1985 (17.6815, 3.1512) -> (17.8817, 3.1037) centre (18.0909, 4.4305) ccw
  arc A1986 (17.8817, 3.1037) -> (18.1619, 3.0725) centre (18.363, 6.1553) ccw
  arc A1987 (18.1619, 3.0725) -> (18.6554, 3.045) centre (19.8494, 28.9382) ccw
  arc A1988 (18.6554, 3.045) -> (19.3062, 3.0215) centre (20.1679, 35.8447) ccw
  arc A1989 (19.3062, 3.0215) -> (19.5062, 3.0541) centre (19.3204, 3.564) ccw
  arc A1990 (19.5062, 3.0541) -> (19.6135, 3.1584) centre (19.4436, 3.2258) ccw
  arc A1991 (19.6135, 3.1584) -> (19.6939, 3.4234) centre (18.0633, 3.7735) ccw
  line L576 (19.6939, 3.4234) -> (19.7358, 3.6184)
  line L577 (19.7358, 3.6184) -> (19.2469, 3.6184)
  arc A1992 (18.934, 3.6211) -> (19.2469, 3.6184) centre (19.2469, 21.976) ccw
  arc A1993 (18.8278, 3.637) -> (18.934, 3.6211) centre (18.941, 4.031) ccw
  arc A1994 (18.7848, 3.6773) -> (18.8278, 3.637) centre (18.8456, 3.699) ccw
  arc A1995 (18.7771, 3.7534) -> (18.7848, 3.6773) centre (18.9352, 3.7309) ccw
  arc A1996 (18.8046, 3.8274) -> (18.7771, 3.7534) centre (18.9604, 3.7274) ccw
  arc A1997 (18.8577, 3.8697) -> (18.8046, 3.8274) centre (18.8935, 3.7703) ccw
  arc A1998 (18.9617, 3.8919) -> (18.8577, 3.8697) centre (18.9912, 3.4992) ccw
  arc A1999 (19.2013, 3.9061) -> (18.9617, 3.8919) centre (19.5392, -3.8079) ccw
  line L578 (19.2013, 3.9061) -> (19.6063, 3.9239)
  line L579 (19.6063, 3.9239) -> (19.6063, 4.1311)
  line L580 (19.6063, 4.1311) -> (19.6063, 4.3384)
  line L581 (19.6063, 4.3384) -> (19.1863, 4.3384)
  arc A2000 (19.0209, 4.3426) -> (19.1863, 4.3384) centre (19.1863, 7.6247) ccw
  arc A2001 (18.8863, 4.3555) -> (19.0209, 4.3426) centre (19.0952, 5.8182) ccw
  arc A2002 (18.7857, 4.3741) -> (18.8863, 4.3555) centre (19.0656, 5.6109) ccw
  arc A2003 (18.7663, 4.3984) -> (18.7857, 4.3741) centre (18.7912, 4.3984) ccw
  arc A2004 (18.7845, 4.4221) -> (18.7663, 4.3984) centre (18.7908, 4.3984) ccw
  arc A2005 (18.8713, 4.4409) -> (18.7845, 4.4221) centre (19.023, 3.5303) ccw
  arc A2006 (18.9873, 4.4541) -> (18.8713, 4.4409) centre (19.0569, 3.3274) ccw
  arc A2007 (19.1263, 4.4584) -> (18.9873, 4.4541) centre (19.1263, 2.203) ccw
  line L582 (19.1263, 4.4584) -> (19.4863, 4.4584)
  line L583 (19.4863, 4.4584) -> (19.4863, 4.6684)
  line L584 (19.4863, 4.6684) -> (19.4863, 4.8784)
  line L585 (19.4863, 4.8784) -> (19.1598, 4.8784)
  arc A2008 (19.0321, 4.8828) -> (19.1598, 4.8784) centre (19.1598, 6.746) ccw
  arc A2009 (18.9184, 4.896) -> (19.0321, 4.8828) centre (19.1144, 6.084) ccw
  arc A2010 (18.8282, 4.9149) -> (18.9184, 4.896) centre (19.0918, 5.9467) ccw
  arc A2011 (18.7963, 4.9384) -> (18.8282, 4.9149) centre (18.8413, 4.9662) ccw
  arc A2012 (18.8041, 4.9636) -> (18.7963, 4.9384) centre (18.8111, 4.9476) ccw
  arc A2013 (18.8657, 4.9825) -> (18.8041, 4.9636) centre (18.916, 4.7088) ccw
  arc A2014 (18.9717, 4.9947) -> (18.8657, 4.9825) centre (19.0107, 4.1932) ccw
  arc A2015 (19.1227, 4.9984) -> (18.9717, 4.9947) centre (19.1227, 1.8933) ccw
  line L586 (19.1227, 4.9984) -> (19.4863, 4.9984)
  line L587 (19.4863, 4.9984) -> (19.4863, 5.2984)
  arc A2016 (19.4904, 5.446) -> (19.4863, 5.2984) centre (22.1113, 5.2984) ccw
  arc A2017 (19.5058, 5.5334) -> (19.4904, 5.446) centre (19.8679, 5.4248) ccw
  arc A2018 (19.5339, 5.5807) -> (19.5058, 5.5334) centre (19.6147, 5.5007) ccw
  arc A2019 (19.5763, 5.5984) -> (19.5339, 5.5807) centre (19.5763, 5.5387) ccw
  arc A2020 (19.5763, 5.5984) -> (19.6174, 5.6134) centre (19.5763, 5.6622) ccw
  arc A2021 (19.6174, 5.6134) -> (19.6457, 5.6534) centre (19.5552, 5.6873) ccw
  arc A2022 (19.6457, 5.6534) -> (19.6617, 5.7251) centre (19.3971, 5.7466) ccw
  arc A2023 (19.6617, 5.7251) -> (19.6663, 5.8384) centre (18.2674, 5.8384) ccw
  arc A2024 (19.6663, 5.8384) -> (19.6617, 5.9517) centre (18.2674, 5.8384) ccw
  arc A2025 (19.6617, 5.9517) -> (19.6457, 6.0234) centre (19.3971, 5.9302) ccw
  arc A2026 (19.6457, 6.0234) -> (19.6174, 6.0634) centre (19.5552, 5.9895) ccw
  arc A2027 (19.6174, 6.0634) -> (19.5763, 6.0784) centre (19.5763, 6.0145) ccw
  arc A2028 (19.5345, 6.0946) -> (19.5763, 6.0784) centre (19.5763, 6.1402) ccw
  arc A2029 (19.5063, 6.1379) -> (19.5345, 6.0946) centre (19.6044, 6.1709) ccw
  arc A2030 (19.4906, 6.2167) -> (19.5063, 6.1379) centre (19.8031, 6.2379) ccw
  arc A2031 (19.4863, 6.3454) -> (19.4906, 6.2167) centre (21.3836, 6.3454) ccw
  line L588 (19.4863, 6.3454) -> (19.4863, 6.6124)
  line L589 (19.4863, 6.6124) -> (19.1413, 6.6304)
  arc A2032 (18.9432, 6.6449) -> (19.1413, 6.6304) centre (19.3887, 11.3736) ccw
  arc A2033 (18.851, 6.668) -> (18.9432, 6.6449) centre (18.9726, 6.9576) ccw
  arc A2034 (18.8025, 6.7105) -> (18.851, 6.668) centre (18.8904, 6.7619) ccw
  arc A2035 (18.7771, 6.7834) -> (18.8025, 6.7105) centre (18.9752, 6.8115) ccw
  arc A2036 (18.7771, 6.7834) -> (18.7551, 6.8548) centre (18.5417, 6.75) ccw
  arc A2037 (18.7551, 6.8548) -> (18.7146, 6.8947) centre (18.6777, 6.8168) ccw
  arc A2038 (18.7146, 6.8947) -> (18.6407, 6.9138) centre (18.6281, 6.712) ccw
  arc A2039 (18.6407, 6.9138) -> (18.4921, 6.9184) centre (18.4921, 4.5326) ccw
  arc A2040 (18.4921, 6.9184) -> (18.3343, 6.9143) centre (18.4921, 3.9059) ccw
  arc A2041 (18.3343, 6.9143) -> (18.2679, 6.8949) centre (18.3422, 6.7631) ccw
  arc A2042 (18.2679, 6.8949) -> (18.2361, 6.8527) centre (18.3003, 6.8375) ccw
  arc A2043 (18.2361, 6.8527) -> (18.2263, 6.7684) centre (18.5928, 6.7684) ccw
  arc A2044 (18.2172, 6.6851) -> (18.2263, 6.7684) centre (17.8407, 6.7684) ccw
  arc A2045 (18.1873, 6.6428) -> (18.2172, 6.6851) centre (18.1518, 6.6996) ccw
  arc A2046 (18.1256, 6.6229) -> (18.1873, 6.6428) centre (18.117, 6.7552) ccw
  arc A2047 (17.9863, 6.6184) -> (18.1256, 6.6229) centre (17.9863, 8.7765) ccw
  arc A2048 (17.9863, 6.6184) -> (17.8529, 6.6139) centre (17.9863, 4.631) ccw
  arc A2049 (17.8529, 6.6139) -> (17.7887, 6.5952) centre (17.8633, 6.4587) ccw
  arc A2050 (17.7887, 6.5952) -> (17.7569, 6.5565) centre (17.8209, 6.5364) ccw
  arc A2051 (17.7569, 6.5565) -> (17.7463, 6.4872) centre (17.9772, 6.4872) ccw
  arc A2052 (17.7422, 6.4093) -> (17.7463, 6.4872) centre (17.0023, 6.4872) ccw
  arc A2053 (17.7236, 6.3953) -> (17.7422, 6.4093) centre (17.7264, 6.411) ccw
  arc A2054 (17.6896, 6.4122) -> (17.7236, 6.3953) centre (17.7355, 6.4619) ccw
  arc A2055 (17.578, 6.5172) -> (17.6896, 6.4122) centre (23.2232, 12.4095) ccw
  arc A2056 (17.578, 6.5172) -> (17.4771, 6.5998) centre (16.9972, 5.9109) ccw
  arc A2057 (17.4771, 6.5998) -> (17.3823, 6.6475) centre (17.263, 6.2926) ccw
  arc A2058 (17.3823, 6.6475) -> (17.2673, 6.6713) centre (17.2264, 6.1834) ccw
  arc A2059 (17.2673, 6.6713) -> (17.098, 6.6784) centre (17.098, 4.6531) ccw
  arc A2060 (16.9785, 6.6823) -> (17.098, 6.6784) centre (17.098, 8.5091) ccw
  arc A2061 (16.8778, 6.6943) -> (16.9785, 6.6823) centre (17.0406, 7.6315) ccw
  arc A2062 (16.8024, 6.7113) -> (16.8778, 6.6943) centre (17.0103, 7.4568) ccw
  arc A2063 (16.7863, 6.7325) -> (16.8024, 6.7113) centre (16.8083, 6.7325) ccw
  arc A2064 (16.7863, 6.7325) -> (16.7584, 6.778) centre (16.7353, 6.7325) ccw
  arc A2065 (16.7584, 6.778) -> (16.6121, 6.8456) centre (15.7703, 4.8316) ccw
  arc A2066 (16.6121, 6.8456) -> (16.4559, 6.9016) centre (15.9937, 5.366) ccw
  arc A2067 (16.4559, 6.9016) -> (16.3416, 6.9184) centre (16.3416, 6.5218) ccw
  arc A2068 (16.3416, 6.9184) -> (16.3099, 6.8997) centre (16.3416, 6.8823) ccw
  arc A2069 (16.3099, 6.8997) -> (16.2611, 6.8022) centre (17.5976, 6.1938) ccw
  arc A2070 (16.2611, 6.8022) -> (16.2098, 6.6745) centre (17.6568, 6.1668) ccw
  arc A2071 (16.2098, 6.6745) -> (16.1615, 6.5229) centre (18.7765, 5.774) ccw
  arc A2072 (16.978, 6.1961) -> (16.9107, 6.1984) centre (16.9107, 5.2271) ccw